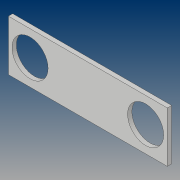
# Autodesk Inventor part: Elasma_diskou2
Saved by Autodesk Inventor 2021 (Build 250183000, 183)
## iProperties
Created: 2020-12-31
Part Number: Elasma_diskou2
Material: Generic
Document SubType Name: Modeling
Designer: Dimitris
Density: 1 g/cm^3
Appearance: Default
Author: Dimitris
Autodesk Inventor part; units mm, degrees
ref_plane "YZ Plane" through (0, 0, 0) normal (1, 0, 0) x (0, 1, 0)
ref_plane "XZ Plane" through (0, 0, 0) normal (0, 1, 0) x (-1, 0, 0)
ref_plane "XY Plane" through (0, 0, 0) normal (0, 0, 1) x (1, 0, 0)
sketch "Sketch1" plane through (0, 0, 0) normal (0, 0, 1) x (1, 0, 0)
  line L0 (-55, 17.5) -> (-55, -17.5)
  line L1 (-55, 17.5) -> (55, 17.5)
  line L2 (55, 17.5) -> (55, -17.5)
  line L3 (55, -17.5) -> (-55, -17.5)
  point P0 (0, 0)
  point P1 (-55, 0)
  dimension "d0" = 35
  dimension "d1" = 55
  dimension "d2" = 110
  dimension "d3" = 35
  constraints: 8 end point, 1 horizontal, 1 horizontal alignment, 1 midpoint, 1 perpendicular, 1 vertical
  measures "d0" distance of L0.start L0.end
  measures "d1" distance of point (0, 0) point (-55, 0)
  measures "d2" distance of L0.start L1.end
  measures "d3" distance of L1.end L2.end
extrude "Extrusion1" add sketch "Sketch1" against normal blind 3
sketch "Sketch2" plane through (0, 0, 0) normal (0, 0, 1) x (1, 0, 0)
  circle A0 centre (40, 0) radius 12.5
  circle A1 centre (-40, 0) radius 12.5
  point P0 (0, 0)
  dimension "d6" = 25
  dimension "d7" = 40
  dimension "d8" = 25
  dimension "d9" = 40
  constraints: 2 centre point, 2 horizontal alignment
  measures "d6" diameter of A0
  measures "d7" distance of point (0, 0) A0.centre
  measures "d8" diameter of A1
  measures "d9" distance of point (0, 0) A1.centre
extrude "Extrusion2" cut sketch "Sketch2" against normal through all
body "Solid1"
